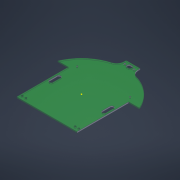
# Autodesk Inventor part: flame
Saved by Autodesk Inventor 2022 (Build 260153000, 153)
## iProperties
Created: 2021-09-22
Part Number: flame
Material: エポキシ樹脂
Document SubType Name: Modeling
Designer: shiok
Density: 1.14 g/cm^3
Appearance: 透明 - スレート 青
Author: shiok
Autodesk Inventor part; units mm, degrees
ref_plane "YZ Plane" through (0, 0, 0) normal (1, 0, 0) x (0, 1, 0)
ref_plane "XZ Plane" through (0, 0, 0) normal (0, 1, 0) x (-1, 0, 0)
ref_plane "XY Plane" through (0, 0, 0) normal (0, 0, 1) x (1, 0, 0)
sketch "スケッチ1" plane through (0, 0, 0) normal (0, 1, 0) x (-1, 0, 0)
  circle A0 centre (0, 0) radius 60
  line L0 (60, 0) -> (-60, 0)
  line L1 (-60, 0) -> (-60, 47)
  line L2 (-60, 47) -> (60, 47)
  line L3 (60, 47) -> (60, 0)
  line L4 (9.5, -70) -> (9.5, -59.2431)
  line L5 (-9.5, -70) -> (-9.5, -59.2431)
  line L6 (9.5, -70) -> (-9.5, -70)
  line L7 (0, -70) -> (0, -60)
  point P0 (37.2961, 47)
  point P1 (3.75, -60.165)
  point P2 (-3.75, -60.165)
  point P3 (-37.2961, 47)
  dimension "d41" = 120
  dimension "d70" = 60.165
  dimension "d71" = 7.5
  dimension "d72" = 3.75
  dimension "d88" = 47
  dimension "d147" = 19
  dimension "d148" = 10
  constraints: 16 end point, 5 point on circle, 3 parallel, 2 coincident, 2 horizontal, 2 midpoint, 1 centre point, 1 horizontal alignment, 1 perpendicular, 1 point on line, 1 vertical, 2 other
  measures "d41" diameter of A0
  measures "d70" vertical distance of point (3.75, -60.165) A0.centre
  measures "d71" distance of point (-3.75, -60.165) point (3.75, -60.165)
  measures "d72" horizontal distance of A0.centre point (3.75, -60.165)
  measures "d88" distance between parallel lines of L0 L2
  measures "d147" distance of L4.start L5.start
  measures "d148" distance of L7.start L7.end
extrude "押し出し1" add sketch "スケッチ1" along normal blind 1.6 contours L0 A0 | L1 L2 A0 | A0 L2 L0 | A0 L7 L6 L5 | A0 L2 L3 | A0 L4 L6 L7
sketch "スケッチ6" plane through (0, 1.6, 0) normal (0, 1, 0) x (-1, 0, 0)
  line L0 (-33.4, -30) -> (-33.4, 42) construction
  line L1 (-33.4, 42) -> (-38.4, 42) construction
  line L2 (-38.4, 42) -> (-38.4, -30) construction
  line L3 (-33.4, 12) -> (-38.4, 12) construction
  line L4 (-40.9, 21.5) -> (-40.9, -18.5) construction
  line L5 (-33.4, -30) -> (-38.4, -30) construction
  line L6 (-42.5, 20) -> (-42.5, -20) construction
  point P0 (0, 0)
  point P1 (-35.9, 0)
  dimension "d52" = 5
  dimension "d53" = 72
  dimension "d54" = 30
  dimension "d55" = 2.5
  dimension "d68" = 33.4
  dimension "d69" = 12
  dimension "d100" = 30
  constraints: 14 end point, 2 point on line, 1 horizontal, 1 parallel, 1 perpendicular
  measures "d52" distance of L1.end L0.end
  measures "d53" distance of L0.end L0.start
  measures "d54" distance between parallel lines of L1 L3
  measures "d55" distance between parallel lines of L2 L4
  measures "d68" distance from line of point (0, 0) L0
  measures "d69" distance from line of point (0, 0) L3
  measures "d100" distance from line of L5 point (-35.9, 0)
hole "穴3" at (33.4, 1.6, 42) at (38.4, 1.6, 42) at (38.4, 1.6, -30) at (33.4, 1.6, -30) at (35.9, 1.6, 0) direction (0, -1, 0) diameter 2.4 end through all clearance for "Countersunk Flat Head Screw ISO 2009/7046" size "M2" standard "ISO"
mirror "ミラー2" about plane through (0, 0, 0) normal (1, 0, 0) of "穴3"
sketch "スケッチ9" plane through (0, 1.6, 0) normal (0, 1, 0) x (1, 0, 0)
  line L0 (-40.9, 23) -> (-70.9, 23)
  line L1 (-70.9, 23) -> (-70.9, -32)
  line L2 (-70.9, -32) -> (-40.9, -32)
  line L3 (-40.9, -32) -> (-40.9, 23)
  line L4 (-60, 0) -> (-60, -47) projected
  line L5 (-60, -47) -> (60, -47) projected
  line L6 (-40.9, -32) -> (-70.9, -32)
  line L7 (-70.9, -32) -> (-70.9, -49)
  line L8 (-70.9, -49) -> (-40.9, -49)
  line L9 (-40.9, -49) -> (-40.9, -32)
  point P0 (0, 0)
  point P1 (-40.9, -47)
  point P2 (-60, -32)
  dimension "d84" = 55
  dimension "d89" = 23
  dimension "d90" = 40.9
  dimension "d91" = 30
  dimension "d92" = 17
  constraints: 16 end point, 4 parallel, 2 horizontal, 2 perpendicular, 1 collinear
  measures "d84" distance between parallel lines of L0 L2
  measures "d89" distance from line of L0 point (0, 0)
  measures "d90" distance from line of L3 point (0, 0)
  measures "d91" distance of L1.end L2.end
  measures "d92" distance of L7.end L6.end
extrude "押し出し2" cut sketch "スケッチ9" against normal blind 10 contours L3 L2 L1 L0 | L9 L5 L4 L2
mirror "ミラー3" about plane through (0, 0, 0) normal (1, 0, 0) of "押し出し2"
sketch "スケッチ12" plane through (0, 1.6, 0) normal (0, 1, 0) x (1, 0, 0)
  line L0 (-56.8017, 16.1133) -> (59.6732, 16.1133) construction
  line L1 (59.6732, 16.1133) -> (59.6732, -15.1509) construction
  line L2 (59.6732, -15.1509) -> (-56.8017, -15.1509) construction
  line L3 (-56.8017, -15.1509) -> (-56.8017, 16.1133) construction
  point P0 (0, 0)
  constraints: 2 other
sketch "スケッチ13" plane through (0, 1.6, 0) normal (0, 1, 0) x (1, 0, 0)
  point P0 (0, 0)
fillet "フィレット1" radius 10 2 edges at (9.5, 0.8, -59.2431) (-9.5, 0.8, -59.2431)
sketch "スケッチ16" plane through (0, 0, 0) normal (0, -1, 0) x (1, 0, 0)
  circle A0 centre (-35.9, 0) radius 1.2 projected
  line L0 (-33.4, -7.5) -> (-38.4, -7.5)
  line L1 (-38.4, -7.5) -> (-38.4, 7.5)
  line L2 (-38.4, 7.5) -> (-33.4, 7.5)
  line L3 (-33.4, 7.5) -> (-33.4, -7.5)
  line L4 (-33.4, -7.5) -> (-38.4, 7.5) construction
  line L5 (-33.4, 7.5) -> (-38.4, -7.5) construction
  point P0 (0, 0)
  point P1 (-35.9, 0)
  dimension "d120" = 5
  dimension "d121" = 15
  constraints: 12 end point, 3 midpoint, 2 parallel, 1 coincident, 1 horizontal, 1 perpendicular
  measures "d120" distance of L1.end L2.end
  measures "d121" distance of L0.end L1.end
extrude "押し出し4" cut sketch "スケッチ16" against normal blind 10
fillet "フィレット2" radius 2 4 edges at (-33.4, 0.8, -7.5) (-33.4, 0.8, 7.5) (-38.4, 0.8, 7.5) (-38.4, 0.8, -7.5)
mirror "ミラー5" about plane through (0, 0, 0) normal (1, 0, 0) of "押し出し4", "フィレット2"
sketch "スケッチ18" plane through (0, 1.6, 0) normal (0, 1, 0) x (1, 0, 0)
  line L0 (-40.4599, 32.0785) -> (41.2884, 32.0785)
  line L1 (41.2884, 32.0785) -> (41.2884, 27.3835)
  line L2 (41.2884, 27.3835) -> (-40.4599, 27.3835)
  line L3 (-40.4599, 27.3835) -> (-40.4599, 32.0785)
  point P0 (0, 0)
  point P1 (33.4, 30)
  point P2 (38.4, 30)
  point P3 (-33.4, 30)
  point P4 (-38.4, 30)
  constraints: 8 end point, 2 parallel, 1 horizontal, 1 perpendicular
extrude "押し出し6" add sketch "スケッチ18" against normal up to surface (1.6 mm away)
sketch "スケッチ19" plane through (0, 1.6, 0) normal (0, 1, 0) x (1, 0, 0)
  line L0 (35.9, 28.75) -> (-35.9, 28.75)
  line L1 (-35.9, 28.75) -> (-35.9, 31.25)
  line L2 (-35.9, 31.25) -> (35.9, 31.25)
  line L3 (35.9, 31.25) -> (35.9, 28.75)
  line L4 (35.9, 30) -> (-35.9, 30)
  line L5 (40.9, 23) -> (55.4166, 23) projected
  line L6 (0, 31.25) -> (0, 28.75)
  point P0 (0, 0)
  point P1 (0, 30)
  dimension "d133" = 7
  dimension "d134" = 71.8
  dimension "d135" = 2.5
  constraints: 12 end point, 5 midpoint, 2 coincident, 2 parallel, 1 horizontal, 1 perpendicular, 1 point on line
  measures "d133" distance between parallel lines of L5 L4
  measures "d134" distance between parallel lines of L1 L3
  measures "d135" distance of L2.end L0.start
hole "穴7" at (35.9, 1.6, -30) at (-35.9, 1.6, -30) direction (0, -1, 0) diameter 1.567 depth 1.6 thread size "M2x0.4" class "6H" standard "ISO Metric profile"
sketch "スケッチ21" plane through (0, 1.6, 0) normal (0, 1, 0) x (1, 0, 0)
  line L0 (9.5, 72.5) -> (-9.5, 72.5) projected
  line L1 (-9.5, 70) -> (9.5, 70)
  line L2 (9.5, 70) -> (9.5, 60)
  line L3 (9.5, 60) -> (-9.5, 60)
  line L4 (-9.5, 60) -> (-9.5, 70)
  line L5 (0, 70) -> (0, 67.5)
  line L6 (-3.1667, 67.5) -> (0, 67.5)
  line L7 (0, 62.5) -> (-3.1667, 62.5)
  line L8 (-3.1667, 62.5) -> (-3.1667, 67.5)
  circle A0 centre (-6.3333, 65) radius 1.5833
  line L9 (0, 65) -> (-1.5833, 65) construction
  line L10 (-1.5833, 65) -> (-3.1667, 65) construction
  line L11 (-3.1667, 65) -> (-4.75, 65) construction
  line L12 (-4.75, 65) -> (-6.3333, 65) construction
  line L13 (-6.3333, 65) -> (-7.9167, 65) construction
  line L14 (-7.9167, 65) -> (-9.5, 65) construction
  line L15 (3.1667, 67.5) -> (0, 67.5)
  line L16 (0, 62.5) -> (3.1667, 62.5)
  line L17 (3.1667, 62.5) -> (3.1667, 67.5)
  circle A1 centre (6.3333, 65) radius 1.5833
  line L18 (0, 65) -> (0, 62.5)
  line L19 (0, 67.5) -> (0, 65)
  line L20 (0, 62.5) -> (0, 60)
  point P0 (0, 0)
  dimension "d146" = 10
  constraints: 40 end point, 8 collinear, 7 parallel, 4 horizontal, 4 midpoint, 3 horizontal alignment, 3 symmetric about line, 2 centre point, 2 point on circle, 1 perpendicular, 1 point on line, 1 vertical alignment, 1 other
  measures "d146" distance of L0.start L2.end
extrude "押し出し7" cut sketch "スケッチ21" against normal blind 1.6 contours L19 L18 L7 L8 L6 | L15 L17 L16 L18 L19
sketch "スケッチ22" plane through (0, 1.6, 0) normal (0, 1, 0) x (1, 0, 0)
  line L0 (-3.1667, 67.5) -> (-3.1667, 62.5) projected
  line L1 (-3.1667, 65) -> (-9.5, 65)
  line L2 (-9.5, 70) -> (-9.5, 67.2291) projected
  line L3 (-3.1667, 67.5) -> (3.1667, 67.5) projected
  line L4 (0, 67.5) -> (0, 65.9167)
  point P0 (0, 0)
  point P1 (-6.3333, 65)
  point P2 (6.3333, 65)
  constraints: 4 end point, 3 midpoint, 1 perpendicular, 1 point on line, 1 symmetric about line, 1 vertical
hole "穴8" at (-6.3333, 1.6, -65) at (6.3333, 1.6, -65) direction (0, -1, 0) diameter 2.4 end through all clearance for "Countersunk Flat Head Screw ISO 2009/7046" size "M2" standard "ISO"
fillet "フィレット5" radius 1.5 4 edges at (-3.1667, 0.8, -67.5) (-3.1667, 0.8, -62.5) (3.1667, 0.8, -62.5) (3.1667, 0.8, -67.5)
